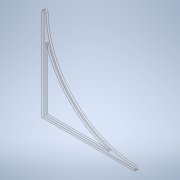
# Autodesk Inventor part: IndexCurveRail
Saved by Autodesk Inventor 2022 (Build 260153000, 153)
## iProperties
Created: 2022-01-14
Part Number: IndexCurveRail
Material: Polycarbonate, Clear
Document SubType Name: Modeling
Designer: tagaz
Density: 1.2 g/cm^3
Appearance: Polycarbonate - Clear
Author: tagaz
Autodesk Inventor part; units mm, degrees
ref_plane "YZ Plane" through (0, 0, 0) normal (1, 0, 0) x (0, 1, 0)
ref_plane "XZ Plane" through (0, 0, 0) normal (0, 1, 0) x (-1, 0, 0)
ref_plane "XY Plane" through (0, 0, 0) normal (0, 0, 1) x (1, 0, 0)
sketch "Sketch1" plane through (0, 0, 0) normal (0, 0, 1) x (1, 0, 0)
  arc A0 (-38.1, 0) -> (0, -38.1) centre (0, 0) ccw
  arc A1 (-266.6279, -6.2023) -> (-6.2023, -266.6279) centre (0, 0) ccw
  line L0 (0, 0) -> (-38.1, 0)
  line L1 (0, 0) -> (0, -38.1)
  arc A2 (-266.7, -83.2795) -> (-83.2795, -266.7) centre (0, 0) ccw
  line L2 (-279.4, -6.35) -> (-279.4, -279.4)
  line L3 (-279.4, -279.4) -> (-6.35, -279.4)
  line L4 (0, -272.9762) -> (0, -273.05)
  line L5 (-272.9762, 0) -> (-273.05, 0)
  line L6 (-83.2795, -266.7) -> (-266.7, -266.7)
  line L7 (-266.7, -266.7) -> (-266.7, -83.2795)
  arc A3 (-266.6279, -6.2023) -> (-272.9762, 0) centre (-272.9762, -6.35) ccw
  arc A4 (-273.05, 0) -> (-279.4, -6.35) centre (-273.05, -6.35) ccw
  arc A5 (0, -272.9762) -> (-6.2023, -266.6279) centre (-6.35, -272.9762) ccw
  arc A6 (-6.35, -279.4) -> (0, -273.05) centre (-6.35, -273.05) ccw
  point P0 (-266.7, 0)
  point P1 (0, -266.7)
  dimension "d0" = 76.2
  dimension "d1" = 228.6
  dimension "d2" = 12.7
  dimension "d3" = 6.35
  dimension "d4" = 6.35
  dimension "d5" = 273.05
  dimension "d6" = 273.05
  constraints: 16 end point, 16 point on circle, 12 tangent, 7 centre point, 5 perpendicular, 2 equal radius, 2 point on line, 1 coincident, 1 horizontal, 1 parallel, 1 vertical
  measures "d0" diameter of A0
  measures "d1" radial gap between concentric circles of A0 A1
  measures "d2" radial gap between concentric circles of A1 A2
  measures "d3" radius of A3
  measures "d4" radius of A5
  measures "d5" distance from line of L3 A4.centre
  measures "d6" distance from line of A6.centre L2
extrude "Extrusion1" add sketch "Sketch1" against normal blind 6.35 contours A1 A5 L4 A6 L3 L2 A4 L5 A3
fillet "Fillet1" radius 0.635 18 edges at (-1.808, -268.5385, -6.35) (0, -273.0131, -6.35) (-1.8599, -277.5401, -6.35) (-142.875, -279.4, -6.35) (-268.5385, -1.808, -6.35) (-273.0131, 0, -6.35) (-277.5401, -1.8599, -6.35) (-279.4, -142.875, -6.35) (-188.5854, -188.5854, -6.35) (-268.5385, -1.808, 0) (-273.0131, 0, 0) (-277.5401, -1.8599, 0) (-279.4, -142.875, 0) (-1.808, -268.5385, 0) (0, -273.0131, 0) (-1.8599, -277.5401, 0) (-142.875, -279.4, 0) (-188.5854, -188.5854, 0)
fillet "Fillet2" radius 0.635 6 edges at (-197.5656, -197.5656, 0) (-174.9897, -266.7, 0) (-266.7, -174.9897, 0) (-266.7, -174.9897, -6.35) (-174.9897, -266.7, -6.35) (-197.5656, -197.5656, -6.35)
body "Solid1"
